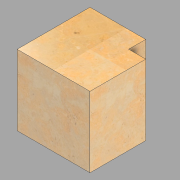
# Autodesk Inventor part: 1-32
Saved by Autodesk Inventor 2022.2 (Build 262287000, 287)
## iProperties
Created: 2021-12-23
Part Number: 1-32
Material: Limestone
Document SubType Name: Modeling
Designer: awelt
Density: 2.6 g/cm^3
Appearance: Amber Select
Mass: 19971.9 g
Surface Area: 2380.44 cm^2
Volume: 7681.5 cm^3
Author: awelt
Autodesk Inventor part; units mm, degrees
ref_plane "YZ Plane" through (0, 0, 0) normal (1, 0, 0) x (0, 1, 0)
ref_plane "XZ Plane" through (0, 0, 0) normal (0, 1, 0) x (-1, 0, 0)
ref_plane "XY Plane" through (0, 0, 0) normal (0, 0, 1) x (1, 0, 0)
sketch "Sketch1" plane through (0, 0, 0) normal (0, 1, 0) x (-1, 0, 0)
  line L0 (101.6, -101.6) -> (-101.6, -101.6)
  line L1 (-101.6, -101.6) -> (-101.6, 101.6)
  line L2 (-101.6, 101.6) -> (101.6, 101.6)
  line L3 (101.6, 101.6) -> (101.6, -101.6)
  line L4 (101.6, -101.6) -> (-101.6, 101.6) construction
  line L5 (-101.6, -101.6) -> (101.6, 101.6) construction
  point P0 (0, 0)
  dimension "d0" = 203.2
  dimension "d1" = 203.2
  constraints: 12 end point, 2 midpoint, 2 parallel, 1 horizontal, 1 perpendicular
  measures "d0" distance of L1.end L2.end
  measures "d1" distance of L0.end L1.end
extrude "Extrusion1" add sketch "Sketch1" along normal blind 196.85
sketch "Sketch2" plane through (0, 196.85, 0) normal (0, 1, 0) x (1, 0, 0)
  line L0 (101.6, -101.6) -> (101.6, 101.6) projected
  line L1 (101.6, 101.6) -> (53.975, 101.6)
  line L2 (53.975, 101.6) -> (53.975, 53.975)
  line L3 (53.975, 53.975) -> (101.6, 53.975)
  line L4 (101.6, 53.975) -> (101.6, 101.6)
  point P0 (0, 0)
  point P1 (101.6, 53.975)
  dimension "d4" = 47.625
  dimension "d5" = 47.625
  constraints: 8 end point, 2 parallel, 1 horizontal, 1 perpendicular
  measures "d4" distance of L3.end L2.end
  measures "d5" distance of L2.end L1.end
extrude "Extrusion2" cut sketch "Sketch2" against normal up to surface (196.85 mm away)
body "Solid1"
